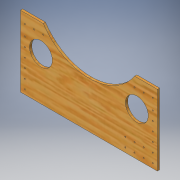
# Autodesk Inventor part: Devant - Bas Rammasse-Balle
Saved by Autodesk Inventor 2016 (Build 200138000, 138)
## iProperties
Created: 2016-01-24
Part Number: Devant - Bas Rammasse-Balle
Material: Generic
Document SubType Name: Modeling
Designer: ares-b02
Density: 1 g/cm^3
Appearance: Plywood - New
Author: ares-b02
Autodesk Inventor part; units mm, degrees
ref_plane "YZ Plane" through (0, 0, 0) normal (1, 0, 0) x (0, 1, 0)
ref_plane "XZ Plane" through (0, 0, 0) normal (0, 1, 0) x (-1, 0, 0)
ref_plane "XY Plane" through (0, 0, 0) normal (0, 0, 1) x (1, 0, 0)
sketch "Sketch1" plane through (0, 0, 0) normal (0, 0, 1) x (1, 0, 0)
  line L0 (186.7379, 130.6481) -> (186.7379, -66.2019)
  line L1 (186.7379, -66.2019) -> (-194.2621, -66.2019)
  line L2 (-194.2621, -66.2019) -> (-194.2621, 130.6481)
  line L3 (-194.2621, 130.6481) -> (-130.7621, 130.6481)
  line L4 (186.7379, 130.6481) -> (123.2379, 130.6481)
  arc A0 (-130.7621, 130.6481) -> (123.2379, 130.6481) centre (-3.7621, 214.8904) ccw
  point P0 (0, 0)
  dimension "d0" = 381
  dimension "d1" = 196.85
  dimension "d41" = 63.5
  dimension "d42" = 63.5
  dimension "d43" = 152.4
  constraints: 10 end point, 2 horizontal, 2 point on circle, 1 centre point, 1 parallel
  measures "d0" distance of L2.end L0.start
  measures "d1" distance of L1.end L2.end
  measures "d41" distance of L0.start L4.end
  measures "d42" distance of L2.end L3.end
  measures "d43" radius of A0
extrude "Extrusion1" add sketch "Sketch1" along normal blind 6.35
hole "Hole2" at (-137.1121, 54.4481, 6.35) direction (0, 0, -1) diameter 63.5 end through all
hole "Hole3" at (129.5879, 54.4481, 6.35) direction (0, 0, -1) diameter 63.5 end through all
hole "Hole4" at (-181.5621, -53.5019, 6.35) direction (0, 0, -1) diameter 3.175 end through all
hole "Hole5" at (174.0379, -53.5019, 6.35) direction (0, 0, -1) diameter 3.175 end through all
pattern_linear "Rectangular Pattern4" count 6 spacing 25.4 along (0, 1, 0) of "Hole4"
pattern_linear "Rectangular Pattern5" count 6 spacing 25.4 along (0, 1, 0) of "Hole5"
pattern_linear "Rectangular Pattern6" count 4 spacing 25.4 along (-1, 0, 0) count 2 spacing 25.4 along (0, 1, 0) of "Hole5"
hole "Hole6" at (-181.5621, 103.6479, 6.35) direction (0, 0, -1) diameter 3.175 end through all
pattern_linear "Rectangular Pattern7" count 20 spacing 25.4 along (1, 0, 0) of "Hole6" skipped copies 4 12
body "Solid1"
